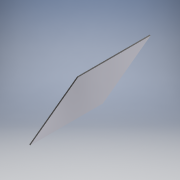
# Autodesk Inventor part: Cabin Back Panel
Saved by Autodesk Inventor 2019 (Build 230136000, 136)
## iProperties
Created: 2019-08-28
Part Number: Cabin Back Panel
Material: Steel, Mild
Document SubType Name: Modeling
Designer: DIBYOJYOTI
Density: 7.85 g/cm^3
Appearance: Semi-Polished
Mass: 62.782 g
Surface Area: 163.565 cm^2
Volume: 7.9977 cm^3
Author: DIBYOJYOTI
Autodesk Inventor part; units mm, degrees
ref_plane "YZ Plane" through (0, 0, 0) normal (1, 0, 0) x (0, 1, 0)
ref_plane "XZ Plane" through (0, 0, 0) normal (0, 1, 0) x (-1, 0, 0)
ref_plane "XY Plane" through (0, 0, 0) normal (0, 0, 1) x (1, 0, 0)
sketch "Sketch1" plane through (0, 0, 0) normal (0, 0, 1) x (1, 0, 0)
  line L0 (133.0032, 6.0018) -> (134.0032, 6.0018)
  line L1 (134.0032, 6.0018) -> (133.0032, 6.0018)
  line L2 (133.0032, -35.2018) -> (81.7369, -124.0001)
  line L3 (81.7369, -124.0001) -> (82.6029, -124.5001)
  line L4 (82.6029, -124.5001) -> (133.8692, -35.7018)
  line L5 (133.8692, -35.7018) -> (133.0032, -35.2018)
  point P0 (0, 0)
  dimension "d0" = 1
  dimension "d1" = 1
  dimension "d4" = 102.5347
  constraints: 12 end point, 2 perpendicular, 1 collinear, 1 horizontal
  measures "d0" distance of L0.start L0.end
  measures "d1" distance of L2.end L3.end
  measures "d4" distance of L3.end L4.end
extrude "Extrusion1" add sketch "Sketch1" along normal blind 78
body "Solid1"
